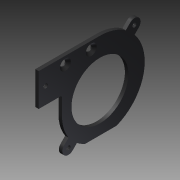
# Autodesk Inventor part: D-005
Saved by Autodesk Inventor 2015 (Build 190159000, 159)
## iProperties
Company: MARCHA TECHNOLOGY
Created: 2014-01-21
Part Number: D-005
Document SubType Name: Modeling
Designer: O.Martin
Density: 7.85 g/cm^3
Project: WITBOXprinter_K01
Stock Number: 2014000004
Material: Steel
Description: SOPORTE FAN BLOWER
Mass: 23.7361 g
Surface Area: 37.6884 cm^2
Volume: 3.0237 cm^3
Appearance: Rubber - Black - Version 1.1
Author: O.Martin
Autodesk Inventor part; units mm, degrees
ref_plane "YZ Plane" through (0, 0, 0) normal (1, 0, 0) x (0, 1, 0)
ref_plane "XZ Plane" through (0, 0, 0) normal (0, 1, 0) x (-1, 0, 0)
ref_plane "XY Plane" through (0, 0, 0) normal (0, 0, 1) x (1, 0, 0)
sketch "Boceto1" plane through (0, 0, 0) normal (0, 0, 1) x (1, 0, 0)
  line L0 (-25.5137, 28.6879) -> (-25.5137, -32.8121)
  line L1 (-25.5137, 28.6879) -> (-23.5137, 28.6879)
  line L2 (-23.5137, 28.6879) -> (-23.5137, -32.8121)
  line L3 (-23.5137, -32.8121) -> (-25.5137, -32.8121)
  dimension "d1" = 2
  dimension "d8" = 61.5
  constraints: 8 end point, 2 perpendicular, 1 horizontal, 1 vertical
  measures "d1" distance of L0.start L1.end
  measures "d8" distance of L0.start L0.end
extrude "Extrusión1" add sketch "Boceto1" along normal mid plane 65
sketch "Boceto2" plane through (-25.5137, -32.8121, 32.5) normal (-1, 0, 0) x (0, 0, 1)
  circle A0 centre (-27.5, 35.5) radius 16.5
  circle A1 centre (-4.6, 55.6) radius 2 projected
  circle A2 centre (-47.2, 17.2) radius 2 projected
  arc A3 (-42.0824, 17.3417) -> (-29.6, 13.5) centre (-29.6, 35.7) ccw projected
  line L0 (-20, 13.5) -> (-29.6, 13.5) projected
  arc A4 (-19, 12.5) -> (-20, 13.5) centre (-20, 12.5) ccw projected
  line L1 (-19, 10.4) -> (-19, 12.5) projected
  line L2 (0, 10.4) -> (-19, 10.4) projected
  line L3 (0, 35.5) -> (0, 10.4) projected
  arc A5 (0, 35.5) -> (-4.7686, 50.5076) centre (-26, 35.5) ccw projected
  line L4 (-2.1374, 53.1129) -> (-4.7686, 50.5076) projected
  arc A6 (-2.1374, 53.1129) -> (-7.0626, 58.0871) centre (-4.6, 55.6) ccw projected
  line L5 (-9.5443, 55.6298) -> (-7.0626, 58.0871) projected
  arc A7 (-9.5443, 55.6298) -> (-26, 61.5) centre (-26, 35.5) ccw projected
  arc A8 (-26, 61.5) -> (-51.8, 35.7) centre (-26, 35.7) ccw projected
  arc A9 (-51.8, 35.7) -> (-47.1808, 22.1444) centre (-29.6, 35.7) ccw projected
  line L6 (-49.6626, 19.6871) -> (-47.1808, 22.1444) projected
  arc A10 (-49.6626, 19.6871) -> (-44.7374, 14.7129) centre (-47.2, 17.2) ccw projected
  line L7 (-42.0824, 17.3417) -> (-44.7374, 14.7129) projected
  line L8 (-65, 0) -> (0, 0) projected
  line L9 (-19, 10.4) -> (-19, 0)
  line L10 (-65, 61.5) -> (-65, 0) projected
  line L11 (0, 10.4) -> (0, 0)
  line L12 (0, 0) -> (-19, 0)
  circle A11 centre (-4.6, 55.6) radius 1
  circle A12 centre (-47.2, 17.2) radius 1
  dimension "d52" = 33
  dimension "d53" = 2
  constraints: 6 end point, 3 centre point, 2 coincident, 1 collinear, 1 equal radius, 1 parallel, 1 perpendicular, 1 point on line
  measures "d52" diameter of A0
  measures "d53" diameter of A12
extrude "Extrusión2" cut sketch "Boceto2" against normal through all contours A1 | A2 | L7 A10 L6 A9 A8 A7 L5 A6 L4 A5 L3 L2 L1 A4 L0 A3 | L2 L11 L8 L9 keep common part
sketch "Boceto3" plane through (-25.5137, -32.8121, 32.5) normal (-1, 0, 0) x (0, 0, 1)
  arc A0 (-2.1374, 53.1129) -> (-7.0626, 58.0871) centre (-4.6, 55.6) ccw projected
  arc A1 (-49.6626, 19.6871) -> (-44.7374, 14.7129) centre (-47.2, 17.2) ccw projected
  constraints: 2 coincident
hole "Agujero1" at (-25.5137, -15.6121, -14.7) at (-25.5137, 22.7879, 27.9) direction (1, 0, 0) diameter 2.459 depth 8 tip angle 118 thread size "M3x0.5" class "6H" standard "ISO Metric profile"
sketch "Boceto4" plane through (-25.5137, -32.8121, 32.5) normal (-1, 0, 0) x (0, 0, 1)
  line L0 (-19, 0) -> (0, 0) projected
  line L1 (-4.5, 10) -> (-4.5, 22.5) construction
  point P0 (-9.5, 4)
  point P1 (-9.5, 0)
  point P2 (-65, 0)
  dimension "d17" = 10
  dimension "d18" = 12.5
  dimension "d26" = 4
  dimension "d54" = 4.5
  constraints: 2 coincident, 2 end point, 1 midpoint, 1 vertical, 1 vertical alignment
  measures "d17" distance from line of L0 L1.start
  measures "d18" distance of L1.start L1.end
  measures "d26" distance from line of L0 point (-9.5, 4)
  measures "d54" distance from line of L0.end L1
hole "Agujero3" at (-25.5137, -28.8121, 23) direction (1, 0, 0) diameter 2.459 end through all thread size "M3x0.5" class "6H" standard "ISO Metric profile"
sketch "Boceto6" plane through (-23.5137, -32.8121, 32.5) normal (1, 0, 0) x (0, 0, -1)
  line L0 (4.5, 15.5) -> (4.5, 30.5) construction
  line L1 (19, 0) -> (0, 0) projected
  line L2 (0, 35.5) -> (0, 0) projected
  dimension "d41" = 15
  dimension "d55" = 4.5
  dimension "d56" = 15.5
  constraints: 2 coincident, 2 end point
  measures "d41" distance of L0.start L0.end
  measures "d55" distance between parallel lines of L2 L0
  measures "d56" distance from line of L1 point (4.5, 15.5)
hole "Agujero5" at (-23.5137, -2.3121, 28) at (-23.5137, -17.3121, 28) direction (-1, 0, 0) diameter 3.4 end through all countersink diameter 6.3 countersink angle 90 clearance for "Tornillo de cabeza avellanada con resalte ISO 2010" size "M3" standard "DIN"
sketch "Boceto7" plane through (-23.5137, -32.8121, 32.5) normal (1, 0, 0) x (0, 0, -1)
  line L0 (0, 35.5) -> (0, 0) projected
  arc A0 (47.1808, 22.1444) -> (51.8, 35.7) centre (29.6, 35.7) ccw projected
  arc A1 (51.8, 35.7) -> (26, 61.5) centre (26, 35.7) ccw projected
  arc A2 (51.8, 35.7) -> (26, 61.5) centre (26, 35.7) ccw projected
  line L1 (50, 45.1678) -> (50, 26.9433)
  arc A3 (47.1808, 22.1444) -> (51.8, 35.7) centre (29.6, 35.7) ccw projected
  dimension "d57" = 50
  constraints: 4 point on circle, 2 end point, 1 vertical
  measures "d57" distance between parallel lines of L1 L0
extrude "Extrusión3" cut sketch "Boceto7" against normal blind 10
body "Solid1"
